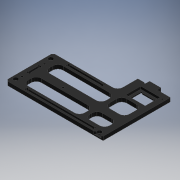
# Autodesk Inventor part: コックピット_2_メインフレーム_1
Saved by Autodesk Inventor 2018 (Build 220112000, 112)
## iProperties
Created: 2016-05-24
Part Number: コックピット_2_メインフレーム_1
Material: アセタール樹脂、黒
Document SubType Name: Modeling
Designer: hiroaki
Density: 1.425 g/cm^3
Appearance: 滑らか - 黒
Mass: 30.4121 g
Surface Area: 156.453 cm^2
Volume: 21.3418 cm^3
d0: 1.000 ul
d1: 0.050 mm
d2: 2.100 mm
d3: 2.100 mm
d4: 0.050 mm
d5: 0.050 mm
d6: 5.000 mm
d7: 0.00 deg
d8: 26.000 mm
d9: 20.000 mm
d10: 3.500 mm
d11: 0.00 deg
d12: 27.000 mm
d13: 43.400 mm
d14: 4.700 mm
d16: 2.500 mm
d20: 2.500 mm
d23: 5.000 mm
d24: 8.000 mm
d25: 5.000 mm
d26: 5.000 mm
d27: 5.000 mm
d28: 4.000 mm
d29: 0.050 mm
d30: 5.000 mm
d31: 10.000 mm
d32: 0.00 deg
d33: 7.000 mm
d34: 2.400 mm
d35: 7.000 mm
d36: 7.000 mm
d37: 60.000 mm
Author: hiroaki
Autodesk Inventor part; units mm, degrees
ref_plane "YZ Plane" through (0, 0, 0) normal (1, 0, 0) x (0, 1, 0)
ref_plane "XZ Plane" through (0, 0, 0) normal (0, 1, 0) x (-1, 0, 0)
ref_plane "XY Plane" through (0, 0, 0) normal (0, 0, 1) x (1, 0, 0)
derived "コックピット_2_基礎_1.ipt"
sketch "スケッチ1" plane through (0, 0, 0) normal (0, 0, 1) x (1, 0, 0)
  line L0 (52.75, 63.5) -> (67.75, 63.5)
  line L1 (67.75, 63.5) -> (67.75, 58.5)
  line L2 (52.75, 63.5) -> (52.75, 58.5)
  line L3 (69.85, 58.5) -> (85.45, 58.5)
  line L4 (85.45, 58.5) -> (85.45, -31.5)
  line L5 (85.45, -31.5) -> (-42.05, -31.5)
  line L6 (-42.05, -31.5) -> (-42.05, 31.5) construction
  line L7 (-42.05, 31.5) -> (42.05, 31.5)
  line L8 (42.05, 31.5) -> (42.05, 58.5)
  line L9 (42.05, 58.5) -> (50.65, 58.5)
  arc A0 (50.65, 58.5) -> (52.75, 58.5) centre (51.7, 58.5) ccw
  arc A1 (67.75, 58.5) -> (69.85, 58.5) centre (68.8, 58.5) ccw
  circle A2 centre (-22.05, 0) radius 1.55
  circle A3 centre (70.45, 0) radius 1.55
  line L10 (-42.05, 31.5) -> (-37.05, 31.5) construction
  line L11 (-37.05, 31.5) -> (-37.05, -31.5) construction
  line L12 (-37.05, -31.5) -> (-42.05, -31.5) construction
  line L13 (-42.05, -31.5) -> (-42.05, 31.5) construction
  circle A4 centre (-39.55, 23.5) radius 1.55
  line L14 (-37.05, 2.5) -> (85.45, 2.5) construction
  line L15 (85.45, 2.5) -> (85.45, -2.5) construction
  line L16 (85.45, -2.5) -> (-37.05, -2.5) construction
  line L17 (-37.05, -2.5) -> (-37.05, 2.5) construction
  line L18 (-37.05, -31.5) -> (85.45, -31.5) construction
  line L19 (85.45, -31.5) -> (85.45, -26.5) construction
  line L20 (85.45, -26.5) -> (-37.05, -26.5) construction
  line L21 (-37.05, -26.5) -> (-37.05, -31.5) construction
  line L22 (-37.05, 31.5) -> (42.05, 31.5) construction
  line L23 (42.05, 31.5) -> (42.05, 26.5) construction
  line L24 (42.05, 26.5) -> (-37.05, 26.5) construction
  line L25 (-37.05, 26.5) -> (-37.05, 31.5) construction
  line L26 (-37.05, 8.5) -> (-39.55, 8.5) construction
  line L27 (-39.55, 8.5) -> (-39.55, -8.5) construction
  line L28 (-39.55, -8.5) -> (-37.05, -8.5) construction
  line L29 (-37.05, -8.5) -> (-37.05, 8.5) construction
  circle A5 centre (-39.55, -23.5) radius 1.55
  line L30 (-42.05, 0) -> (-53.9458, 0) construction
  line L31 (-42.05, 31.5) -> (-44.55, 29)
  line L32 (-44.55, 29) -> (-44.55, -29)
  line L33 (-44.55, -29) -> (-42.05, -31.5)
  line L34 (-22.05, -26.5) -> (70.45, -26.5) construction
  line L35 (70.45, -26.5) -> (70.45, -29) construction
  line L36 (70.45, -29) -> (-22.05, -29) construction
  line L37 (-22.05, -29) -> (-22.05, -26.5) construction
  line L38 (-22.05, 26.5) -> (27.05, 26.5) construction
  line L39 (27.05, 26.5) -> (27.05, 29) construction
  line L40 (27.05, 29) -> (-22.05, 29) construction
  line L41 (-22.05, 29) -> (-22.05, 26.5) construction
  circle A6 centre (-39.55, 23.5) radius 3 construction
  line L42 (55.65, 48.5) -> (75.25, 48.5)
  line L43 (75.25, 48.5) -> (75.25, 35.4)
  line L44 (75.25, 35.4) -> (55.65, 35.4)
  line L45 (55.65, 35.4) -> (55.65, 48.5)
  line L46 (-30.05, 23.5) -> (45.95, 23.5)
  line L47 (45.95, 23.5) -> (45.95, 5.5)
  line L48 (45.95, 5.5) -> (-30.05, 5.5)
  line L49 (-30.05, 5.5) -> (-30.05, 23.5)
  line L50 (-30.05, -5.5) -> (45.95, -5.5)
  line L51 (45.95, -5.5) -> (45.95, -23.5)
  line L52 (45.95, -23.5) -> (-30.05, -23.5)
  line L53 (-30.05, -23.5) -> (-30.05, -5.5)
  circle A7 centre (-22.05, 0) radius 3 construction
  line L54 (-39.6, 8.55) -> (-37, 8.55)
  line L55 (-37, 8.55) -> (-37, -8.55)
  line L56 (-37, -8.55) -> (-39.6, -8.55)
  line L57 (-39.6, -8.55) -> (-39.6, 8.55)
  circle A8 centre (-39.6, 7.5) radius 1.05
  circle A9 centre (-37, 7.5) radius 1.05
  circle A10 centre (-39.6, -7.5) radius 1.05
  circle A11 centre (-37, -7.5) radius 1.05
  line L58 (-22.1, -26.45) -> (70.5, -26.45)
  line L59 (70.5, -26.45) -> (70.5, -29.05)
  line L60 (70.5, -29.05) -> (-22.1, -29.05)
  line L61 (-22.1, -29.05) -> (-22.1, -26.45)
  circle A12 centre (-21.05, -26.45) radius 1.05
  circle A13 centre (-21.05, -29.05) radius 1.05
  circle A14 centre (69.45, -26.45) radius 1.05
  circle A15 centre (69.45, -29.05) radius 1.05
  circle A16 centre (56.7, 48.5) radius 1.05
  circle A17 centre (74.2, 48.5) radius 1.05
  circle A18 centre (74.2, 35.4) radius 1.05
  circle A19 centre (56.7, 35.4) radius 1.05
  line L62 (-22.1, 29.05) -> (27.1, 29.05)
  line L63 (27.1, 29.05) -> (27.1, 26.45)
  line L64 (27.1, 26.45) -> (-22.1, 26.45)
  line L65 (-22.1, 26.45) -> (-22.1, 29.05)
  circle A20 centre (-21.05, 29.05) radius 1.05
  circle A21 centre (-21.05, 26.45) radius 1.05
  circle A22 centre (26.05, 29.05) radius 1.05
  circle A23 centre (26.05, 26.45) radius 1.05
  circle A24 centre (-38.05, -16.5) radius 1.2
  circle A25 centre (1.95, -1.5) radius 1.2
  circle A26 centre (-38.05, 13.5) radius 1.2
  line L66 (-29.05, -23.5) -> (28.95, -23.5) construction
  line L67 (-26.55, -23.5) -> (23.45, -23.5) construction
  line L68 (23.45, -23.5) -> (23.45, -16.5) construction
  line L69 (23.45, -16.5) -> (-26.55, -16.5) construction
  line L70 (-26.55, -16.5) -> (-26.55, -23.5) construction
  circle A27 centre (81.95, 51.5) radius 1.2
  circle A28 centre (81.95, 51.5) radius 3.5 construction
  circle A29 centre (81.95, -8.5) radius 1.2
  line L71 (21.7, -31.5) -> (21.7, 31.5) construction
  circle A30 centre (77.95, -29) radius 1.55
  point P0 (0, 0)
  point P1 (0, 31.5)
  point P2 (-39.55, 31.5)
  point P3 (-44.55, 0)
  point P4 (-37.05, -29)
  point P5 (-37.05, 29)
  point P6 (65.45, 48.5)
  point P7 (60.25, 63.5)
  dimension "d2" = 2.1
  dimension "d3" = 2.1
  dimension "d1" = 0.05
  dimension "d4" = 0.05
  dimension "d5" = 0.05
  dimension "d34" = 2.4
  dimension "d35" = 7
  dimension "d36" = 7
  dimension "d37" = 60
  measures "d1" distance between parallel lines of L54 L26
  measures "d4" distance between parallel lines of L58 L34
  measures "d5" distance between parallel lines of L62 L40
  measures "d34" diameter of A27
  measures "d35" diameter of A28
  measures "d36" distance from line of L3 A27.centre
  measures "d37" distance of A29.centre A27.centre
extrude "押し出し1" add sketch "スケッチ1" along normal blind 5 contours L0 L1 A1 L3 L4 L5 L33 L32 L31 L7 L8 L9 A0 L2 | A2 | A3 | A24 | A26 | A29
sketch "スケッチ3" plane through (-42.05, -31.5, 5) normal (0, 0, 1) x (1, 0, 0)
  line L0 (115.2, 66.9) -> (99.8, 66.9) projected
  arc A0 (97.7, 66.9) -> (99.8, 66.9) centre (98.75, 66.9) ccw projected
  line L1 (97.7, 66.9) -> (97.7, 80) projected
  arc A1 (99.8, 80) -> (97.7, 80) centre (98.75, 80) ccw projected
  line L2 (99.8, 80) -> (115.2, 80) projected
  arc A2 (117.3, 80) -> (115.2, 80) centre (116.25, 80) ccw projected
  line L3 (117.3, 80) -> (117.3, 66.9) projected
  arc A3 (115.2, 66.9) -> (117.3, 66.9) centre (116.25, 66.9) ccw projected
  line L4 (120.5, 83.45) -> (94.5, 83.45)
  line L5 (94.5, 83.45) -> (94.5, 63.45)
  line L6 (94.5, 63.45) -> (120.5, 63.45)
  line L7 (120.5, 63.45) -> (120.5, 83.45)
  circle A4 centre (2.5, 8) radius 1.55 projected
  circle A5 centre (2.5, 55) radius 1.55 projected
  circle A6 centre (2.5, 55) radius 3
  circle A7 centre (2.5, 8) radius 3
  circle A8 centre (120, 2.5) radius 1.55 projected
  circle A9 centre (120, 2.5) radius 3
  point P0 (42.05, 31.5)
  point P1 (107.5, 63.45)
  point P2 (107.5, 66.9)
  point P3 (120.5, 73.45)
  point P4 (117.3, 73.45)
  point P5 (112.5, 31.5)
  point P6 (20, 31.5)
  dimension "d8" = 26
  dimension "d9" = 20
  dimension "d39" = 6
  dimension "d40" = 6
  constraints: 8 end point, 4 coincident, 4 midpoint, 3 centre point, 2 parallel, 1 equal radius, 1 horizontal, 1 horizontal alignment, 1 perpendicular, 1 vertical alignment
  measures "d8" distance of L5.end L6.end
  measures "d9" distance of L6.end L4.start
  measures "d39" diameter of A6
  measures "d40" diameter of A9
extrude "押し出し2" cut sketch "スケッチ3" against normal blind 3.5
sketch "スケッチ4" plane through (42.05, 58.5, 0) normal (0, 1, 0) x (1, 0, 0)
  line L0 (0, 0) -> (0, -5) projected
  line L1 (43.4, 0) -> (43.4, -5) projected
  point P0 (-42.05, 0)
  point P1 (4.7, -2.5)
  point P2 (31.7, -2.5)
  point P3 (0, -2.5)
  dimension "d12" = 27
  dimension "d13" = 43.4
  dimension "d14" = 4.7
  constraints: 2 horizontal alignment, 1 midpoint
  measures "d12" distance of point (31.7, -2.5) point (4.7, -2.5)
  measures "d13" distance between parallel lines of L1 L0
  measures "d14" distance from line of L0 point (4.7, -2.5)
hole "穴1" at (46.75, 58.5, 2.5) at (73.75, 58.5, 2.5) direction (0, -1, 0) diameter 2.459 depth 2.5 thread size "M3x0.5" class "6H" standard "ISO Metric profile"
sketch "スケッチ5" plane through (-42.05, -31.5, 5) normal (0, 0, 1) x (1, 0, 0)
  line L0 (120.5, 63.45) -> (94.5, 63.45) projected
  circle A0 centre (112.5, 31.5) radius 3 projected
  line L1 (88, 55) -> (88, 37) projected
  line L2 (88, 26) -> (88, 8) projected
  line L3 (110.45, 2.45) -> (22.05, 2.45) projected
  arc A1 (19.95, 2.45) -> (22.05, 2.45) centre (21, 2.45) ccw projected
  line L4 (19.95, 2.45) -> (19.95, 5.05) projected
  arc A2 (22.05, 5.05) -> (19.95, 5.05) centre (21, 5.05) ccw projected
  line L5 (22.05, 5.05) -> (110.45, 5.05) projected
  arc A3 (112.55, 5.05) -> (110.45, 5.05) centre (111.5, 5.05) ccw projected
  line L6 (112.55, 5.05) -> (112.55, 2.45) projected
  arc A4 (110.45, 2.45) -> (112.55, 2.45) centre (111.5, 2.45) ccw projected
  line L7 (127.5, 0) -> (127.5, 90) projected
  line L8 (93, 59.45) -> (119.5, 59.45)
  line L9 (119.5, 59.45) -> (119.5, 36.5)
  line L10 (119.5, 36.5) -> (93, 36.5)
  line L11 (93, 36.5) -> (93, 59.45)
  line L12 (93, 26.5) -> (119.5, 26.5)
  line L13 (119.5, 26.5) -> (119.5, 10)
  line L14 (119.5, 10) -> (93, 10)
  line L15 (93, 10) -> (93, 26.5)
  line L16 (110.5013, 5) -> (21.9987, 5)
  arc A5 (21.9987, 5) -> (20, 5.05) centre (21, 5.05) ccw
  line L17 (20, 5.05) -> (20, 2.45)
  arc A6 (20, 2.45) -> (21.9987, 2.5) centre (21, 2.45) ccw
  line L18 (21.9987, 2.5) -> (110.5013, 2.5)
  arc A7 (110.5013, 2.5) -> (112.5, 2.45) centre (111.5, 2.45) ccw
  line L19 (112.5, 2.45) -> (112.5, 5.05)
  arc A8 (112.5, 5.05) -> (110.5013, 5) centre (111.5, 5.05) ccw
  point P0 (42.05, 31.5)
  dimension "d23" = 5
  dimension "d24" = 8
  dimension "d25" = 5
  dimension "d26" = 5
  dimension "d27" = 5
  dimension "d28" = 4
  dimension "d29" = 0.05
  dimension "d30" = 5
  constraints: 24 end point, 8 point on circle, 4 centre point, 4 parallel, 2 horizontal, 2 perpendicular, 1 vertical alignment, 7 other
  measures "d23" distance between parallel lines of L11 L1
  measures "d24" distance between parallel lines of L7 L9
  measures "d25" distance from line of A0.centre L10
  measures "d26" distance from line of L12 A0.centre
  measures "d27" distance between parallel lines of L2 L15
  measures "d28" distance between parallel lines of L0 L8
  measures "d29" distance between parallel lines of L5 L16
  measures "d30" distance between parallel lines of L14 L16
extrude "押し出し3" cut sketch "スケッチ5" against normal blind 10 contours L8 L9 L10 L11 | L12 L13 L14 L15
fillet "フィレット1" radius 7 17 edges at (50.95, 5, 2.5) (45.95, 5.5, 2.5) (50.95, -5, 2.5) (45.95, -5.5, 2.5) (77.45, -5, 2.5) (77.45, 5, 2.5) (77.45, 27.95, 2.5) (50.95, 27.95, 2.5) (45.95, 23.5, 2.5) (-30.05, 23.5, 2.5) (-30.05, 5.5, 2.5) (-30.05, -5.5, 2.5) (-30.05, -23.5, 2.5) (45.95, -23.5, 2.5) (50.95, -21.5, 2.5) (77.45, -21.5, 2.5) (42.05, 31.5, 2.5)
fillet "フィレット1" radius 2 2 edges at (76.2917, -31.5, 3.25) (79.6083, -31.5, 3.25)
equation "\"d26\" = d25"
equation "\"d27\" = d23"
